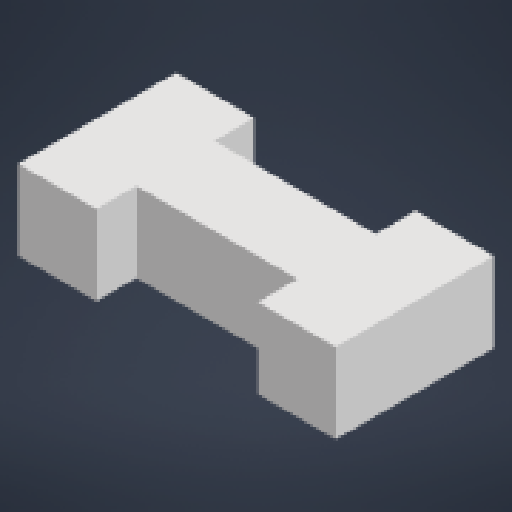
# Autodesk Inventor part: 5mm_pin
Saved by Autodesk Inventor 2026 (Build 300175050, 175E)
## iProperties
Created: 2026-04-30
Part Number: 5mm_pin
Material: Generic
Document SubType Name: Modeling
Designer: sniel
Density: 1 g/cm^3
Appearance: Default
Author: sniel
Autodesk Inventor part; units mm, degrees
ref_plane "YZ Plane" through (0, 0, 0) normal (1, 0, 0) x (0, 1, 0)
ref_plane "XZ Plane" through (0, 0, 0) normal (0, 1, 0) x (-1, 0, 0)
ref_plane "XY Plane" through (0, 0, 0) normal (0, 0, 1) x (1, 0, 0)
sketch "Sketch1" plane through (0, 0, 0) normal (0, 1, 0) x (-1, 0, 0)
  line L0 (0, 0) -> (-5, 0)
  line L1 (5, 0) -> (0, 0)
  line L2 (-5, 0) -> (-5, 2.5)
  line L3 (-5, 2.5) -> (-10, 2.5)
  line L4 (-10, 2.5) -> (-10, -7.5)
  line L5 (-10, -7.5) -> (-5, -7.5)
  line L6 (-5, -7.5) -> (-5, -5)
  line L7 (-5, -5) -> (0, -5)
  line L8 (0, -5) -> (5, -5)
  line L9 (5, 2.5) -> (5, 0)
  line L10 (10, 2.5) -> (5, 2.5)
  line L11 (10, -7.5) -> (10, 2.5)
  line L12 (5, -5) -> (5, -7.5)
  line L13 (5, -7.5) -> (10, -7.5)
  line L14 (-10, 2.5) -> (-9.95, 2.5)
  line L15 (-9.95, 2.5) -> (-9.95, 2.45)
  line L16 (-9.95, 2.45) -> (-10, 2.45)
  line L17 (-10, 2.45) -> (-10, 2.5)
  line L18 (-5, 2.5) -> (-5.05, 2.5)
  line L19 (-5.05, 2.5) -> (-5.05, 2.45)
  line L20 (-5.05, 2.45) -> (-5, 2.45)
  line L21 (-5, 2.45) -> (-5, 2.5)
  line L22 (-10, -7.5) -> (-9.95, -7.5)
  line L23 (-9.95, -7.5) -> (-9.95, -7.45)
  line L24 (-9.95, -7.45) -> (-10, -7.45)
  line L25 (-10, -7.45) -> (-10, -7.5)
  line L26 (-5, -7.5) -> (-5.05, -7.5)
  line L27 (-5.05, -7.5) -> (-5.05, -7.45)
  line L28 (-5.05, -7.45) -> (-5, -7.45)
  line L29 (-5, -7.45) -> (-5, -7.5)
  line L30 (-5, 0) -> (-5.05, 0)
  line L31 (-5.05, 0) -> (-5.05, -0.05)
  line L32 (-5.05, -0.05) -> (-5, -0.05)
  line L33 (-5, -0.05) -> (-5, 0)
  line L34 (10, -7.5) -> (9.95, -7.5)
  line L35 (9.95, -7.5) -> (9.95, -7.45)
  line L36 (9.95, -7.45) -> (10, -7.45)
  line L37 (10, -7.45) -> (10, -7.5)
  line L38 (5, 2.5) -> (5.05, 2.5)
  line L39 (5.05, 2.5) -> (5.05, 2.45)
  line L40 (5.05, 2.45) -> (5, 2.45)
  line L41 (5, 2.45) -> (5, 2.5)
  line L42 (5, -5) -> (5.05, -5)
  line L43 (5.05, -5) -> (5.05, -4.95)
  line L44 (5.05, -4.95) -> (5, -4.95)
  line L45 (5, -4.95) -> (5, -5)
  line L46 (9.95, -7.45) -> (5.05, -7.45)
  line L47 (5.05, -7.45) -> (5.05, 2.45)
  line L48 (5.05, 2.45) -> (9.95, 2.45)
  line L49 (9.95, 2.45) -> (9.95, -7.45)
  line L50 (5.05, -4.95) -> (-5.05, -4.95)
  line L51 (-5.05, -4.95) -> (-5.05, -0.05)
  line L52 (-5.05, -0.05) -> (5.05, -0.05)
  line L53 (5.05, -0.05) -> (5.05, -4.95)
  line L54 (-5.05, 2.45) -> (-9.95, 2.45)
  line L55 (-9.95, 2.45) -> (-9.95, -7.45)
  line L56 (-9.95, -7.45) -> (-5.05, -7.45)
  line L57 (-5.05, -7.45) -> (-5.05, 2.45)
  dimension "d2" = 0.05
  dimension "d3" = 0.05
  dimension "d4" = 0.05
  dimension "d5" = 0.05
  dimension "d6" = 0.05
  dimension "d7" = 0.05
  dimension "d8" = 0.05
  dimension "d9" = 0.05
  dimension "d10" = 0.05
  dimension "d11" = 0.05
  dimension "d12" = 0.05
  dimension "d13" = 0.05
  dimension "d14" = 0.05
  dimension "d15" = 0.05
  dimension "d16" = 0.05
  dimension "d17" = 0.05
  constraints: 116 end point, 22 parallel, 11 horizontal, 11 perpendicular
  measures "d2" distance of L15.end L16.end
  measures "d3" distance of L14.end L15.end
  measures "d4" distance of L20.end L19.end
  measures "d5" distance of L19.end L18.end
  measures "d6" distance of L24.end L23.end
  measures "d7" distance of L23.end L22.end
  measures "d8" distance of L27.end L28.end
  measures "d9" distance of L26.end L27.end
  measures "d10" distance of L32.end L31.end
  measures "d11" distance of L31.end L30.end
  measures "d12" distance of L35.end L36.end
  measures "d13" distance of L34.end L35.end
  measures "d14" distance of L39.end L40.end
  measures "d15" distance of L38.end L39.end
  measures "d16" distance of L44.end L43.end
  measures "d17" distance of L43.end L42.end
extrude "Extrusion1" add sketch "Sketch1" along normal blind 5
body "Solid1"
